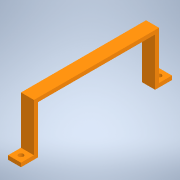
# Autodesk Inventor part: battery_pack_clamp_v2
Saved by Autodesk Inventor 2020.3 (Build 243373000, 373)
## iProperties
Created: 2020-11-24
Part Number: battery_pack_clamp_v2
Material: PET Plastic
Document SubType Name: Modeling
Designer: Devin
Density: 1.541 g/cm^3
Appearance: Orange
Author: Devin
Autodesk Inventor part; units mm, degrees
ref_plane "YZ Plane" through (0, 0, 0) normal (1, 0, 0) x (0, 1, 0)
ref_plane "XZ Plane" through (0, 0, 0) normal (0, 1, 0) x (-1, 0, 0)
ref_plane "XY Plane" through (0, 0, 0) normal (0, 0, 1) x (1, 0, 0)
sketch "Sketch1" plane through (0, 0, 0) normal (1, 0, 0) x (0, 1, 0)
  line L0 (0.0837, -1.2362) -> (0.0837, -73.5362)
  line L1 (0.0837, -73.5362) -> (-29.4163, -73.5362)
  line L2 (-29.4163, -1.2362) -> (0.0837, -1.2362)
  line L3 (2.4837, -75.9362) -> (2.4837, 1.1638)
  line L4 (2.4837, 1.1638) -> (-27.0163, 1.1638)
  line L5 (-27.0163, -75.9362) -> (2.4837, -75.9362)
  line L6 (-27.0163, 1.1638) -> (-27.0163, 9.1638)
  line L7 (-27.0163, 9.1638) -> (-29.4163, 9.1638)
  line L8 (-27.0163, -75.9362) -> (-27.0163, -83.9362)
  line L9 (-27.0163, -83.9362) -> (-29.4163, -83.9362)
  line L10 (-29.4163, 9.1638) -> (-29.4163, -1.2362)
  line L11 (-29.4163, -73.5362) -> (-29.4163, -83.9362)
  point P0 (0, 0)
  dimension "d10" = 29.5
  dimension "d11" = 72.3
  dimension "d12" = 2.4
  dimension "d13" = 2.4
  dimension "d14" = 2.4
  dimension "d15" = 2.4
  dimension "d16" = 2.4
  dimension "d17" = 8
  dimension "d25" = 8
  constraints: 24 end point, 4 parallel, 2 perpendicular, 2 vertical, 1 horizontal
  measures "d10" distance between parallel lines of L10 L0
  measures "d11" distance between parallel lines of L1 L2
  measures "d12" distance between parallel lines of L5 L1
  measures "d13" distance between parallel lines of L4 L2
  measures "d14" distance between parallel lines of L3 L0
  measures "d15" distance between parallel lines of L11 L8
  measures "d16" distance between parallel lines of L10 L6
  measures "d17" distance between parallel lines of L7 L4
  measures "d25" distance between parallel lines of L5 L9
extrude "Extrusion1" add sketch "Sketch1" along normal blind 8
sketch "Sketch2" plane through (0, -27.0163, 9.1638) normal (0, 1, 0) x (1, 0, 0)
  line L0 (0, 8) -> (8, 8) projected
  line L1 (8, 8) -> (8, 0) projected
  line L2 (0, 8) -> (8, 8) projected
  line L3 (0, 0) -> (8, 0) projected
  circle A0 centre (4, 4) radius 1.5
  line L4 (0, 93.1) -> (0, 85.1) projected
  circle A1 centre (4, 89.1) radius 1.5
  point P0 (0, 9.1638)
  point P1 (8, 93.1)
  point P2 (8, 85.1)
  dimension "d26" = 3
  dimension "d27" = 3
  constraints: 2 centre point
  measures "d26" diameter of A0
  measures "d27" diameter of A1
extrude "Extrusion2" cut sketch "Sketch2" against normal blind 10
body "Solid1"
